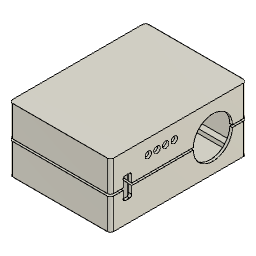
AQS-Simple-Case-v5 (Autodesk Fusion 360 design; units mm, degrees)
Autodesk Fusion 360 part; units mm, degrees
sketch "Sketch1" plane through (0, 0, 0) normal (0, 0, 1) x (1, 0, 0)
  line L0 (19.2, -25.3) -> (-19.2, -25.3)
  line L1 (-19.2, -25.3) -> (-19.2, 25.3)
  line L2 (-19.2, 25.3) -> (19.2, 25.3)
  line L3 (19.2, 25.3) -> (19.2, -25.3)
  line L4 (19.2, -25.3) -> (-19.2, 25.3) construction
  line L5 (-19.2, -25.3) -> (19.2, 25.3) construction
  line L6 (20.4, -26.5) -> (-20.4, -26.5)
  line L7 (-20.4, -26.5) -> (-20.4, 26.5)
  line L8 (-20.4, 26.5) -> (20.4, 26.5)
  line L9 (20.4, 26.5) -> (20.4, -26.5)
  line L10 (20.4, -26.5) -> (-20.4, 26.5) construction
  line L11 (-20.4, -26.5) -> (20.4, 26.5) construction
  line L12 (-20.4, -26.5) -> (20.4, -26.5)
  line L13 (20.4, -26.5) -> (20.4, -36.5)
  line L14 (20.4, -36.5) -> (-20.4, -36.5)
  line L15 (-20.4, -36.5) -> (-20.4, -26.5)
  line L16 (-20.4, 26.5) -> (-26.4, 26.5)
  line L17 (-26.4, 26.5) -> (-26.4, -36.5)
  line L18 (-26.4, -36.5) -> (-20.4, -36.5)
  line L19 (-20.4, -36.5) -> (-20.4, 26.5)
  line L20 (-19.2, 25.3) -> (-25.2, 25.3)
  line L21 (-25.2, 25.3) -> (-25.2, -35.3)
  line L22 (-25.2, -35.3) -> (19.2, -35.3)
  line L23 (19.2, -35.3) -> (19.2, -25.3)
  dimension "d1" = 38.4
  dimension "d2" = 50.6
  dimension "d3" = 40.8
  dimension "d4" = 53
  dimension "d5" = 10
  dimension "d6" = 6
  dimension "d7" = 1.2
  dimension "d8" = 1.2
  constraint perpendicular L0 L1
  constraint parallel L0 L2
  constraint parallel L1 L3
  constraint horizontal L0
  constraint coincident L4 origin
  constraint coincident L5 origin
  constraint perpendicular L6 L7
  constraint parallel L6 L8
  constraint parallel L7 L9
  constraint horizontal L6
  constraint coincident L10 origin
  constraint coincident L11 origin
  constraint horizontal L12
  constraint vertical L13
  constraint horizontal L14
  constraint vertical L15
  constraint horizontal L16
  constraint vertical L17
  constraint horizontal L18
  constraint vertical L19
  constraint coincident L14.end L15.start
  constraint perpendicular L7 L20
  constraint perpendicular L20 L21
  constraint perpendicular L21 L22
  constraint parallel L13 L23
  measures "d1" distance of L1.end L2.end
  measures "d2" distance of L0.end L1.end
  measures "d3" distance of L7.end L8.end
  measures "d4" distance of L6.end L7.end
  measures "d5" distance of L6.end L14.end
  measures "d6" distance of L7.end L16.end
  measures "d7" distance of L17 L21
  measures "d8" distance of L14 L22
  measures "d15" distance of L0.start
extrude "Extrude1" add sketch "Sketch1" along normal blind 13 contours L2 L3 L6 L7 L8 L9 L12 L19 L20 L23 | L6 L12 L13 L14 L15 L19 L22 L23 | L7 L15 L16 L17 L18 L19 L20 L21 L22 makes body 1
extrude "Extrude2" add sketch "Sketch1" against normal blind 1.2 bodies 1
extrude "Extrude3" add sketch "Sketch1" along normal blind 13 contours L0 L1 L6 L7 L12 L19 L20 L23 bodies 1
sketch "Sketch2" plane through (0, 0, 13) normal (0, 0, 1) x (-1, 0, 0)
  line L0 (-19.2, 26.5) -> (-19.2, 35.3)
  line L1 (-19.2, 35.3) -> (25.2, 35.3)
  line L2 (25.2, 35.3) -> (25.2, -25.3)
  line L3 (25.2, -25.3) -> (20.4, -25.3)
  line L4 (-20.4, -26.5) -> (26.4, -26.5)
  line L5 (26.4, -26.5) -> (26.4, 36.5)
  line L6 (26.4, 36.5) -> (-20.4, 36.5)
  line L7 (-20.4, 36.5) -> (-20.4, -26.5)
  line L8 (20.4, -19.3) -> (19.2, -19.3)
  line L9 (19.2, -19.3) -> (19.2, -3.3)
  line L10 (19.2, -3.3) -> (20.4, -3.3)
  line L11 (20.4, -3.3) -> (20.4, -19.3)
  line L12 (19.2, -25.3) -> (-19.2, -25.3)
  line L13 (20.4, -25.3) -> (20.4, 26.5)
  line L14 (20.4, 26.5) -> (-19.2, 26.5)
  line L15 (-19.2, 25.3) -> (19.2, 25.3)
  line L16 (19.2, 25.3) -> (19.2, -25.3)
  line L17 (19.2, -25.3) -> (-19.2, -25.3)
  line L18 (-19.2, -25.3) -> (-19.2, 25.3)
  dimension "d15" = 6
  dimension "d16" = 16
  constraint horizontal L8
  constraint vertical L9
  constraint horizontal L10
  constraint vertical L11
  measures "d15" distance of L8 L12
  measures "d16" distance of L8.end L9.end
extrude "Extrude4" cut sketch "Sketch2" against normal blind 5 contours L8 L9 L10 L11 L13 L16 bodies 1
sketch "Sketch3" plane through (20.4, 0, 0) normal (1, 0, 0) x (0, 1, 0)
  line L0 (26.5, -1.2) -> (26.5, 13)
  line L1 (26.5, 13) -> (-36.5, 13)
  line L2 (-36.5, 13) -> (-36.5, -1.2)
  line L3 (-36.5, -1.2) -> (26.5, -1.2)
  circle A0 centre (10.8, 13) radius 9
  line L4 (25.3, 0) -> (25.3, 13)
  dimension "d19" = 18
  dimension "d20" = 14.5
  constraint coincident L1 A0.centre
  measures "d19" diameter of A0
  measures "d20" distance of A0.centre L4
extrude "Extrude5" cut sketch "Sketch3" against normal up to surface (1.2 mm away) contours L1 A0 picked at (10.5758, 10.0084) bodies 1
sketch "Sketch4" plane through (0, 0, 0) normal (0, 0, 1) x (1, 0, 0)
  line L0 (-19.2, 25.3) -> (19.2, 25.3)
  line L1 (19.2, 25.3) -> (19.2, 22.5)
  line L2 (19.2, 22.5) -> (-19.2, 22.5)
  line L3 (-19.2, 22.5) -> (-19.2, 25.3)
  line L4 (-19.2, -25.3) -> (19.2, -25.3)
  line L5 (19.2, -25.3) -> (19.2, -22.5)
  line L6 (19.2, -22.5) -> (-19.2, -22.5)
  line L7 (-19.2, -22.5) -> (-19.2, -25.3)
  point P0 (-19.2, -25.3)
  point P1 (19.2, -25.3)
  point P2 (-19.2, 25.3)
  point P3 (19.2, 25.3)
  constraint horizontal L0
  constraint vertical L1
  constraint horizontal L2
  constraint vertical L3
  constraint horizontal L4
  constraint vertical L5
  constraint horizontal L6
  constraint vertical L7
  constraint coincident P0 L4.start
  constraint coincident P1 L4.end
  constraint coincident P2 L0.start
  constraint coincident P3 L0.end
extrude "Extrude6" add sketch "Sketch4" along normal blind 2 bodies 1
sketch "Sketch5" plane through (0, 0, 0) normal (0, 0, 1) x (-1, 0, 0)
  line L0 (-19.2, 26.5) -> (20.4, 26.5)
  line L1 (20.4, 26.5) -> (20.4, -25.3)
  line L2 (20.4, -25.3) -> (25.2, -25.3)
  line L3 (25.2, -25.3) -> (25.2, 35.3)
  line L4 (25.2, 35.3) -> (-19.2, 35.3)
  line L5 (-19.2, 35.3) -> (-19.2, 26.5)
  line L6 (-19.2, 31.1926) -> (15.8, 31.1926)
  line L7 (15.8, 31.1926) -> (15.8, 29.9926)
  line L8 (15.8, 29.9926) -> (-19.2, 29.9926)
  line L9 (-19.2, 29.9926) -> (-19.2, 31.1926)
  line L10 (-19.2, 31.1926) -> (15.8, 29.9926) construction
  line L11 (15.8, 31.1926) -> (-19.2, 29.9926) construction
  line L12 (-19.2, 32.3926) -> (15.8, 32.3926)
  line L13 (15.8, 32.3926) -> (15.8, 28.7926)
  line L14 (15.8, 28.7926) -> (-19.2, 28.7926)
  line L15 (-19.2, 28.7926) -> (-19.2, 32.3926)
  line L16 (-19.2, 32.3926) -> (15.8, 28.7926) construction
  line L17 (15.8, 32.3926) -> (-19.2, 28.7926) construction
  line L18 (17, 26.5) -> (15.8, 26.5)
  line L19 (15.8, 26.5) -> (15.8, 35.3)
  line L20 (15.8, 35.3) -> (17, 35.3)
  line L21 (17, 35.3) -> (17, 26.5)
  point P0 (-1.7, 30.5926)
  point P1 (-1.7, 30.5926)
  dimension "d25" = 35
  dimension "d26" = 1.2
  dimension "d27" = 3.6
  dimension "d28" = 1.2
  constraint perpendicular L6 L7
  constraint parallel L6 L8
  constraint parallel L7 L9
  constraint horizontal L6
  constraint coincident L10 P1
  constraint coincident L11 P1
  constraint collinear L5 L9
  constraint perpendicular L12 L13
  constraint parallel L12 L14
  constraint parallel L13 L15
  constraint horizontal L12
  constraint coincident L16 P1
  constraint coincident L17 P1
  constraint coincident P1 P0
  constraint horizontal L18
  constraint vertical L19
  constraint horizontal L20
  constraint vertical L21
  constraint coincident L4 L19.end
  constraint coincident L0 L18.start
  constraint collinear L13 L19
  measures "d25" distance of L7.end L8.end
  measures "d26" distance of L6.end L7.end
  measures "d27" distance of L12.end L13.end
  measures "d28" distance of L19 L21
extrude "Extrude7" add sketch "Sketch5" along normal blind 5 contours L0 L4 L7 L13 L18 L19 L20 L21 bodies 1
extrude "Extrude8" add sketch "Sketch5" along normal blind 0.8 contours L5 L8 L13 L14 L15 L19 | L5 L6 L12 L13 L15 L19 bodies 1
sketch "Sketch6" plane through (0, 0, 0.8) normal (0, 0, 1) x (-1, 0, 0)
  line L0 (15.8, 29.9926) -> (-19.2, 29.9926)
  line L1 (-19.2, 29.9926) -> (-19.2, 28.7926)
  line L2 (-19.2, 28.7926) -> (15.8, 28.7926)
  line L3 (15.8, 28.7926) -> (15.8, 29.9926)
  line L4 (-19.2, 28.7926) -> (-13.2, 28.7926)
  line L5 (-13.2, 28.7926) -> (-13.2, 29.9926)
  line L6 (-13.2, 29.9926) -> (-19.2, 29.9926)
  line L7 (-19.2, 29.9926) -> (-19.2, 28.7926)
  line L8 (-19.2, 32.3926) -> (-13.2, 32.3926)
  line L9 (-13.2, 32.3926) -> (-13.2, 31.1926)
  line L10 (-13.2, 31.1926) -> (-19.2, 31.1926)
  line L11 (-19.2, 31.1926) -> (-19.2, 32.3926)
  point P0 (-19.2, 32.3926)
  dimension "d33" = 6
  dimension "d36" = 6
  dimension "d37" = 1.2
  constraint horizontal L4
  constraint vertical L5
  constraint horizontal L6
  constraint vertical L7
  constraint coincident L1.end L2.start
  constraint horizontal L8
  constraint vertical L9
  constraint horizontal L10
  constraint vertical L11
  constraint coincident P0 L8.start
  constraint collinear L0 L6
  measures "d33" distance of L1.end L4.end
  measures "d36" distance of P0 L8.end
  measures "d37" distance of P0 L10.end
extrude "Extrude9" cut sketch "Sketch6" against normal up to surface (0.8 mm away) contours L0 L1 L2 L4 L5 L6 L7 bodies 1
extrude "Extrude10" cut sketch "Sketch6" against normal up to surface (0.8 mm away) contours L8 L9 L10 L11 bodies 1
sketch "Sketch7" plane through (20.4, 0, 0) normal (1, 0, 0) x (0, 1, 0)
  arc A0 (1.8, 13) -> (19.8, 13) centre (10.8, 13) ccw
  line L0 (1.8, 13) -> (-36.5, 13)
  line L1 (-36.5, 13) -> (-36.5, -1.2)
  line L2 (-36.5, -1.2) -> (26.5, -1.2)
  line L3 (26.5, -1.2) -> (26.5, 13)
  line L4 (26.5, 13) -> (19.8, 13)
  line L5 (-30.6419, 13) -> (-26.6419, 13)
  line L6 (-26.6419, 13) -> (-26.6419, 8.5)
  line L7 (-26.6419, 8.5) -> (-30.6419, 8.5)
  line L8 (-30.6419, 8.5) -> (-30.6419, 13)
  dimension "d40" = 4
  dimension "d41" = 4.5
  constraint horizontal L5
  constraint vertical L6
  constraint horizontal L7
  constraint vertical L8
  constraint coincident L0 L5.start
  measures "d40" distance of L5.start L5.end
  measures "d41" distance of L5.start L7.end
extrude "Extrude11" cut sketch "Sketch7" against normal up to surface (1.2 mm away) contours L0 L5 L6 L7 L8 bodies 1
fillet "Fillet1" radius 1 2 edges at (19.8, -26.6419, 8.5) (19.8, -30.6419, 8.5) on bodies 1
fillet "Fillet2" radius 1.5 4 edges at (19.2, -35.3, 6.5) (-25.2, -35.3, 6.5) (-25.2, 25.3, 6.5) (19.2, 25.3, 7.5) on bodies 1
fillet "Fillet3" radius 1.5 4 edges at (20.4, 26.5, 5.9) (-26.4, 26.5, 5.9) (-26.4, -36.5, 5.9) (20.4, -36.5, 5.9) on bodies 1
fillet "Fillet4" radius 1.5 8 edges at (-19.2, -25.3, 7.5) (19.2, -25.3, 7.5) (-19.2, 25.3, 7.5) (-20.4, 25.3, 6.5) (-17, -26.5, 2.5) (-15.8, -26.5, 2.5) (-15.8, -35.3, 2.5) (-17, -35.3, 2.5) on bodies 1
fillet "Fillet5" radius 1.5 1 edges at (-20.4, -26.5, 6.5) on bodies 1
fillet "Fillet6" radius 1 1 edges at (19.2, -26.5, 6.5) on bodies 1
fillet "Fillet7" radius 1.5 2 edges at (-19.8, 19.3, 8) (-19.8, 3.3, 8) on bodies 1
delete_face "DeleteFace1" 1 faces at (18.6272, 24.9791, 5.6667) on bodies 1
delete_face "DeleteFace2" 1 faces at (-18.7856, 24.8351, 9.3333) on bodies 1
delete_face "DeleteFace3" 1 faces at (-18.6272, -24.9791, 5.6667) on bodies 1
delete_face "DeleteFace4" 1 faces at (18.6272, -24.9791, 5.6667) on bodies 1
mirror "Mirror1" [no effect]
mirror "Mirror2" about plane through (0, 0, 0) normal (0, 0, 1) of bodies 1 makes body 2
move_body "Move2" bodies 2 to x (1, 0, 0) y (0, 1, 0) z (0, 0, 1) at (0, 0, 27)
sketch "Sketch8" plane through (20.4, 0, 0) normal (1, 0, 0) x (0, 1, 0)
  line L0 (-35, 28.2) -> (-35, 14)
  line L1 (-35, 14) -> (-30.6419, 14)
  line L2 (-30.6419, 14) -> (-30.6419, 17.5)
  arc A0 (-29.6419, 18.5) -> (-30.6419, 17.5) centre (-29.6419, 17.5) ccw
  line L3 (-29.6419, 18.5) -> (-27.6419, 18.5)
  arc A1 (-26.6419, 17.5) -> (-27.6419, 18.5) centre (-27.6419, 17.5) ccw
  line L4 (-26.6419, 17.5) -> (-26.6419, 14)
  line L5 (-26.6419, 14) -> (1.8, 14)
  arc A2 (19.8, 14) -> (1.8, 14) centre (10.8, 14) ccw
  line L6 (19.8, 14) -> (25, 14)
  line L7 (25, 14) -> (25, 28.2)
  line L8 (25, 28.2) -> (-35, 28.2)
  line L9 (27.2295, 21.5) -> (-36.7705, 21.5) construction
  circle A3 centre (-19, 21.5) radius 1.5
  circle A4 centre (-15, 21.5) radius 1.5
  circle A5 centre (-11, 21.5) radius 1.5
  circle A6 centre (-7, 21.5) radius 1.5
  line L10 (-25, 14) -> (-25, 27)
  dimension "d53" = 7.5
  dimension "d54" = 3
  dimension "d55" = 3
  dimension "d56" = 3
  dimension "d57" = 3
  dimension "d58" = 4
  dimension "d59" = 4
  dimension "d60" = 4
  dimension "d61" = 6
  constraint perpendicular L7 L9
  constraint coincident L9 A3.centre
  constraint coincident L9 A4.centre
  constraint coincident L9 A5.centre
  constraint coincident L9 A6.centre
  measures "d53" distance of L5 L9
  measures "d54" diameter of A3
  measures "d55" diameter of A4
  measures "d56" diameter of A5
  measures "d57" diameter of A6
  measures "d58" distance of A5.centre A6.centre
  measures "d59" distance of A4.centre A5.centre
  measures "d60" distance of A3.centre A4.centre
  measures "d61" distance of A3.centre L10
extrude "Extrude12" cut sketch "Sketch8" against normal up to surface (1.2 mm away) contours A3 | A4 | A5 | A6 bodies 2
delete_face "DeleteFace5" 1 faces at (-20, 4.6574, 8.0068) on bodies 1
delete_face "DeleteFace6" 1 faces at (-19.6, 17.9426, 8.0068) on bodies 1
delete_face "DeleteFace7" 1 faces at (-20, 19.3, 9.6667) on bodies 1
sketch "Sketch9" plane through (0, 0, 13) normal (0, 0, 1) x (-1, 0, 0)
  line L0 (24.9, 36.5) -> (-18.9, 36.5)
  arc A0 (-18.9, 36.5) -> (-20.4, 35) centre (-18.9, 35) ccw
  line L1 (-20.4, 35) -> (-20.4, 30.6419)
  line L2 (-20.4, 30.6419) -> (-19.2, 30.6419)
  line L3 (-19.2, 30.6419) -> (-19.2, 33.8)
  arc A1 (-17.7, 35.3) -> (-19.2, 33.8) centre (-17.7, 33.8) ccw
  line L4 (-17.7, 35.3) -> (23.7, 35.3)
  arc A2 (25.2, 33.8) -> (23.7, 35.3) centre (23.7, 33.8) ccw
  line L5 (25.2, 33.8) -> (25.2, -23.8)
  arc A3 (23.7, -25.3) -> (25.2, -23.8) centre (23.7, -23.8) ccw
  line L6 (23.7, -25.3) -> (21.9, -25.3)
  arc A4 (20.4, -23.8) -> (21.9, -25.3) centre (21.9, -23.8) ccw
  line L7 (20.4, -23.8) -> (20.4, 25)
  arc A5 (20.4, 25) -> (18.9, 26.5) centre (18.9, 25) ccw
  line L8 (18.9, 26.5) -> (-18.2, 26.5)
  arc A6 (-18.7135, 26.6419) -> (-18.2, 26.5) centre (-18.2, 27.5) ccw
  line L9 (-18.7135, 26.6419) -> (-20.4, 26.6419)
  line L10 (-20.4, 26.6419) -> (-20.4, -1.8)
  line L11 (-20.4, -1.8) -> (-19.2, -1.8)
  line L12 (-19.2, -1.8) -> (-19.2, 25.3)
  line L13 (-19.2, 25.3) -> (19.2, 25.3)
  line L14 (19.2, 25.3) -> (19.2, -25.3)
  line L15 (19.2, -25.3) -> (-19.2, -25.3)
  line L16 (-19.2, -25.3) -> (-19.2, -19.8)
  line L17 (-19.2, -19.8) -> (-20.4, -19.8)
  line L18 (-20.4, -19.8) -> (-20.4, -25)
  arc A7 (-20.4, -25) -> (-18.9, -26.5) centre (-18.9, -25) ccw
  line L19 (-18.9, -26.5) -> (24.9, -26.5)
  arc A8 (24.9, -26.5) -> (26.4, -25) centre (24.9, -25) ccw
  line L20 (26.4, -25) -> (26.4, 35)
  arc A9 (26.4, 35) -> (24.9, 36.5) centre (24.9, 35) ccw
  line L21 (21, 27) -> (-14, 27)
  line L22 (-14, 27) -> (-14, -20)
  line L23 (-14, -20) -> (21, -20)
  line L24 (21, -20) -> (21, 27)
  constraint horizontal L21
  constraint vertical L22
  constraint horizontal L23
  constraint vertical L24
extrude "Extrude13" cut sketch "Sketch9" against normal blind 5 contours L13 L14 L22 L23 | L7 A5 L8 L13 L14 L22 L23 | L7 A5 L8 L21 L22 L23 L24 bodies 1
fillet "Fillet8" radius 2 2 edges at (-19.8, 20, 8) (14, -25.9, 8) on bodies 1
delete_face "DeleteFace8" 1 faces at (-20, 18.7272, 18.6791) on bodies 2
delete_face "DeleteFace9" 1 faces at (-19.6, 3.501, 18.25) on bodies 2
delete_face "DeleteFace10" 1 faces at (-19.6, 3.3, 17.3333) on bodies 2
sketch "Sketch10" plane through (0, 0, 14) normal (0, 0, -1) x (1, 0, 0)
  line L0 (-20.4, 25) -> (-20.4, -23.8)
  arc A0 (-21.9, -25.3) -> (-20.4, -23.8) centre (-21.9, -23.8) ccw
  line L1 (-21.9, -25.3) -> (-23.7, -25.3)
  arc A1 (-25.2, -23.8) -> (-23.7, -25.3) centre (-23.7, -23.8) ccw
  line L2 (-25.2, -23.8) -> (-25.2, 33.8)
  arc A2 (-23.7, 35.3) -> (-25.2, 33.8) centre (-23.7, 33.8) ccw
  line L3 (-23.7, 35.3) -> (17.7, 35.3)
  arc A3 (19.2, 33.8) -> (17.7, 35.3) centre (17.7, 33.8) ccw
  line L4 (19.2, 33.8) -> (19.2, 30.6419)
  line L5 (19.2, 30.6419) -> (20.4, 30.6419)
  line L6 (20.4, 30.6419) -> (20.4, 35)
  arc A4 (20.4, 35) -> (18.9, 36.5) centre (18.9, 35) ccw
  line L7 (18.9, 36.5) -> (-24.9, 36.5)
  arc A5 (-24.9, 36.5) -> (-26.4, 35) centre (-24.9, 35) ccw
  line L8 (-26.4, 35) -> (-26.4, -25)
  arc A6 (-26.4, -25) -> (-24.9, -26.5) centre (-24.9, -25) ccw
  line L9 (-24.9, -26.5) -> (18.9, -26.5)
  arc A7 (18.9, -26.5) -> (20.4, -25) centre (18.9, -25) ccw
  line L10 (20.4, -25) -> (20.4, -19.8)
  line L11 (20.4, -19.8) -> (19.2, -19.8)
  line L12 (19.2, -19.8) -> (19.2, -25.3)
  line L13 (19.2, -25.3) -> (-19.2, -25.3)
  line L14 (-19.2, -25.3) -> (-19.2, 25.3)
  line L15 (-19.2, 25.3) -> (19.2, 25.3)
  line L16 (19.2, 25.3) -> (19.2, -1.8)
  line L17 (19.2, -1.8) -> (20.4, -1.8)
  line L18 (20.4, -1.8) -> (20.4, 26.6419)
  line L19 (20.4, 26.6419) -> (18.7135, 26.6419)
  arc A8 (18.2, 26.5) -> (18.7135, 26.6419) centre (18.2, 27.5) ccw
  line L20 (18.2, 26.5) -> (-18.9, 26.5)
  arc A9 (-18.9, 26.5) -> (-20.4, 25) centre (-18.9, 25) ccw
  line L21 (-21, 27) -> (14, 27)
  line L22 (14, 27) -> (14, -19)
  line L23 (14, -19) -> (-21, -19)
  line L24 (-21, -19) -> (-21, 27)
  constraint horizontal L21
  constraint vertical L22
  constraint horizontal L23
  constraint vertical L24
extrude "Extrude14" cut sketch "Sketch10" against normal blind 5 contours L0 L14 L15 L20 A9 L22 L23 | L0 L20 A9 L21 L22 L23 L24 | L14 L15 L22 L23 bodies 2
fillet "Fillet9" radius 2 2 edges at (-19.8, 19, 19) (14, -25.9, 19) on bodies 2
sketch "Sketch11" plane through (0, 0, 26.2) normal (0, 0, -1) x (1, 0, 0)
  line L0 (13.2, 28.7926) -> (13.2, 29.9926)
  line L1 (13.2, 29.9926) -> (-15.8, 29.9926)
  line L2 (-15.8, 29.9926) -> (-15.8, 28.7926)
  line L3 (-15.8, 28.7926) -> (13.2, 28.7926)
  line L4 (-10.8, 33) -> (-10.8, 28.3) construction
  line L5 (-15.8, 33.8) -> (-15.8, 28) construction
  line L6 (-15.8, 32.381) -> (-10.8, 32.381)
  line L7 (-10.8, 32.381) -> (-10.8, 31.181)
  line L8 (-10.8, 31.181) -> (-15.8, 31.181)
  line L9 (-15.8, 31.181) -> (-15.8, 32.381)
  line L10 (-15.8, 28.7926) -> (-10.8, 28.7926)
  line L11 (-10.8, 28.7926) -> (-10.8, 29.9926)
  line L12 (-10.8, 29.9926) -> (-15.8, 29.9926)
  line L13 (-15.8, 29.9926) -> (-15.8, 28.7926)
  dimension "d70" = 5
  dimension "d71" = 1.2
  constraint vertical L4
  constraint horizontal L6
  constraint vertical L7
  constraint horizontal L8
  constraint vertical L9
  constraint coincident L5 L6.start
  constraint horizontal L10
  constraint vertical L11
  constraint horizontal L12
  constraint vertical L13
  constraint coincident L4 L11.end
  constraint coincident L1 L11.end
  constraint coincident L2.end L3.start
  measures "d70" distance of L4 L5
  measures "d71" distance of L6.start L8.end
extrude "Extrude15" add sketch "Sketch11" along normal blind 3.2 contours L1 L2 L3 L10 L11 L12 L13 | L6 L7 L8 L9 bodies 2
sketch "Sketch12" plane through (0, 0, 0.8) normal (0, 0, 1) x (-1, 0, 0)
  line L0 (-13.2, 32.3926) -> (-13.2, 31.1926)
  line L1 (-13.2, 31.1926) -> (15.8, 31.1926)
  line L2 (15.8, 31.1926) -> (15.8, 32.3926)
  line L3 (15.8, 32.3926) -> (-13.2, 32.3926)
  line L4 (10.8, 28.4) -> (10.8, 33.1) construction
  line L5 (15.8, 33.8) -> (15.8, 28) construction
  line L6 (15.8, 32.3926) -> (10.8, 32.3926)
  line L7 (10.8, 32.3926) -> (10.8, 31.1926)
  line L8 (10.8, 31.1926) -> (15.8, 31.1926)
  line L9 (15.8, 31.1926) -> (15.8, 32.3926)
  line L10 (15.8, 29.9926) -> (10.8, 29.9926)
  line L11 (10.8, 29.9926) -> (10.8, 28.7926)
  line L12 (10.8, 28.7926) -> (15.8, 28.7926)
  line L13 (15.8, 28.7926) -> (15.8, 29.9926)
  line L14 (15.8, 29.9926) -> (-13.2, 29.9926)
  dimension "d74" = 5
  dimension "d75" = 1.2
  constraint vertical L4
  constraint horizontal L6
  constraint vertical L7
  constraint horizontal L8
  constraint vertical L9
  constraint coincident L1 L7.end
  constraint coincident L4 L7.end
  constraint coincident L2.end L3.start
  constraint horizontal L10
  constraint vertical L11
  constraint horizontal L12
  constraint vertical L13
  constraint coincident L5 L10.start
  constraint collinear L10 L14
  measures "d74" distance of L4 L5
  measures "d75" distance of L10.start L12.end
extrude "Extrude16" add sketch "Sketch12" along normal blind 3.2 contours L1 L2 L3 L6 L7 L8 L9 | L10 L11 L12 L13 L14 bodies 1
move_face "OffsetFaces1" offset -0.2 1 faces at (-14.1333, -29.9926, 1.6) on bodies 1
move_face "OffsetFaces2" offset -0.2 1 faces at (-14.1333, -31.1926, 1.6) on bodies 1
move_face "OffsetFaces3" offset 0.2 1 faces at (-14.1333, -28.7926, 1.6) on bodies 1
move_face "OffsetFaces4" offset 0.2 1 faces at (-14.1333, -32.3926, 1.6) on bodies 1
move_face "OffsetFaces5" offset -0.2158 2 faces at (-14.1333, -29.9926, 25.4) (-12.4667, -31.181, 25.1333) on bodies 2
move_face "OffsetFaces6" offset -0.2 1 faces at (3.5333, -31.1926, 26.7333) on bodies 2
move_face "OffsetFaces7" offset -0.0116 1 faces at (3.5333, -32.3926, 26.7333) on bodies 2
